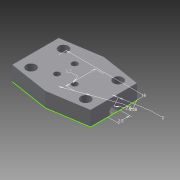
# Autodesk Inventor part: LED cooling tubing cap 2
Saved by Autodesk Inventor 2013 SP2 (Build 170200200, 200)
## iProperties
Created: 2014-12-12
Part Number: LED cooling tubing cap 2
Material: Generic
Document SubType Name: Modeling
Designer: kthorn
Density: 1 g/cm^3
Author: kthorn
Autodesk Inventor part; units mm, degrees
ref_plane "YZ Plane" through (0, 0, 0) normal (1, 0, 0) x (0, 1, 0)
ref_plane "XZ Plane" through (0, 0, 0) normal (0, 1, 0) x (-1, 0, 0)
ref_plane "XY Plane" through (0, 0, 0) normal (0, 0, 1) x (1, 0, 0)
sketch "Sketch1" plane through (0, 0, 0) normal (0, 0, 1) x (1, 0, 0)
  line L0 (-8.0095, -1.25) -> (7.9905, -1.25) construction
  line L1 (7.9905, -1.25) -> (7.9905, 1.25) construction
  line L2 (7.9905, 1.25) -> (-8.0095, 1.25) construction
  line L3 (-8.0095, 1.25) -> (-8.0095, -1.25) construction
  line L4 (-8.0095, -1.25) -> (7.9905, 1.25) construction
  line L5 (7.9905, -1.25) -> (-8.0095, 1.25) construction
  circle A0 centre (5.5829, 3.3205) radius 1
  line L6 (-0.0095, 0) -> (-0.0095, 6) construction
  line L7 (-0.0095, 0) -> (-0.0095, -6) construction
  line L8 (-0.0095, 6) -> (-8.0095, 4.75)
  line L9 (-8.0095, 4.75) -> (-8.0095, -4.75)
  line L10 (-8.0095, -4.75) -> (-0.0095, -6)
  line L11 (-0.0095, 6) -> (7.9905, 4.75)
  line L12 (7.9905, 4.75) -> (7.9905, -4.75)
  line L13 (7.9905, -4.75) -> (-0.0095, -6)
  line L14 (7.9905, 4.75) -> (-8.0095, -4.75) construction
  line L15 (-8.0095, 4.75) -> (7.9905, -4.75) construction
  circle A1 centre (-5.6019, 3.3205) radius 1
  line L16 (-8.0095, 0) -> (7.9905, 0) construction
  circle A2 centre (5.5829, -3.3205) radius 1
  circle A3 centre (-5.6019, -3.3205) radius 1
  circle A4 centre (-0.0095, 0) radius 2.54 construction
  line L17 (-0.0095, 0) -> (1.7866, -1.796) construction
  line L18 (-0.0095, 0) -> (-1.8055, -1.796) construction
  line L19 (-0.0095, 0) -> (-1.8055, 1.7961) construction
  circle A5 centre (1.7866, -1.796) radius 0.6
  circle A6 centre (-1.8055, -1.796) radius 0.6
  circle A7 centre (-1.8055, 1.7961) radius 0.6
  point P0 (0, 0)
  point P1 (-0.0095, 0)
  point P2 (-0.0095, 0)
  dimension "d1" = 2.5
  dimension "d2" = 2
  dimension "d3" = 6
  dimension "d4" = 16
  dimension "d5" = 2.8
  dimension "d13" = 5.08
  dimension "d14" = 1.2
  constraints: 40 end point, 8 centre point, 7 coincident, 6 parallel, 5 equal length, 5 midpoint, 3 perpendicular, 3 point on circle, 3 symmetric about line, 2 equal radius, 2 point on line, 1 collinear, 3 other
  measures "d1" distance of L0.end L2.start
  measures "d2" diameter of A0
  measures "d3" distance of L6.start L11.start
  measures "d4" distance between parallel lines of L12 L9
  measures "d5" distance of L14.start A0.centre
  measures "d13" diameter of A4
  measures "d14" diameter of A7
extrude "Extrusion2" add sketch "Sketch1" along normal blind 3
sketch "Sketch2" plane through (7.9905, -4.75, 0) normal (1, 0, 0) x (0, 0, -1)
  line L0 (0, 9.5) -> (0, 0) projected
  arc A0 (-0.7, 5.6) -> (-0.7, 3.9) centre (-0.7, 4.75) ccw
  line L1 (-0.7, 5.6) -> (0, 5.6)
  line L2 (-0.7, 3.9) -> (0, 3.9)
  line L3 (0, 5.6) -> (0, 3.9)
  line L4 (-3, 0) -> (-3, 9.5) projected
  line L5 (-3, 4.75) -> (-0.7, 4.75) construction
  point P0 (0, 4.75)
  dimension "d11" = 1.7
  dimension "d19" = 0.7
  constraints: 8 end point, 3 perpendicular, 2 point on circle, 2 point on line, 2 tangent, 1 centre point, 1 horizontal, 1 midpoint
  measures "d11" diameter of A0
  measures "d19" distance from line of L0 L5.end
sketch "Sketch3" plane through (0, 0, 0) normal (0, 0, -1) x (-1, 0, 0)
  line L0 (-7.9905, 4.75) -> (-7.9905, -4.75) projected
  line L1 (8.0095, -4.75) -> (8.0095, 4.75) projected
  line L2 (-7.9905, 0) -> (8.0095, 0)
  point P0 (0, 0)
  constraints: 2 end point, 2 midpoint
sweep "Sweep1" cut profiles "Sketch2" path "Sketch3" path curves L2
body "Solid2"
